Autodesk Inventor part; units mm, degrees
(part 2 of 2)
sketch "Sketch20" plane through (0, 0, 1) normal (0, 0, -1) x (-1, 0, 0)
  circle A0 centre (13.284, -4.42) radius 2.05 projected
  circle A1 centre (-13.284, 4.42) radius 2.05 projected
  circle A2 centre (-2.8142, 13.7142) radius 2.05 projected
  circle A3 centre (2.8142, -13.7142) radius 2.05 projected
  circle A4 centre (-10.4698, -9.2943) radius 2.05 projected
  circle A5 centre (10.4698, 9.2943) radius 2.05 projected
  arc A6 (-16.9842, 20.9889) -> (18.8277, -19.3525) centre (0, 0) ccw projected
  line L0 (18.8277, -19.3525) -> (17.641, -18.1327) projected
  arc A7 (16.8781, -10.7298) -> (17.641, -18.1327) centre (21.9416, -13.9488) ccw projected
  arc A8 (16.8781, -10.7298) -> (-8.6535, 18.031) centre (0, 0) ccw projected
  arc A9 (-15.9137, 19.666) -> (-8.6535, 18.031) centre (-11.2495, 23.4403) ccw projected
  line L1 (-15.9137, 19.666) -> (-16.9842, 20.9889) projected
  circle A10 centre (0, 0) radius 8.075 projected
  circle A11 centre (0, 0) radius 20
  circle A12 centre (-25.0527, -22.2399) radius 2.05 projected
  circle A13 centre (-31.7866, 10.5764) radius 2.05 projected
  circle A14 centre (-31.7866, 10.5764) radius 2.05 projected
  line L2 (0, 0) -> (-31.7866, 10.5764)
  circle A15 centre (-25.0527, -22.2399) radius 2.05 projected
  line L3 (0, 0) -> (-25.0527, -22.2399)
  line L4 (0, 0) -> (-25.7367, -8.1623)
  arc A16 (-16.9842, 20.9889) -> (18.8277, -19.3525) centre (0, 0) ccw projected
  point P0 (-25.7367, -8.1623)
  point P1 (-19.0642, -6.0461)
  point P2 (-18.9771, 6.3143)
  point P3 (-25.6191, 8.5242)
  dimension "d87" = 40
  dimension "d88" = 24
  constraints: 6 end point, 1 centre point, 1 coincident, 1 point on circle
  measures "d87" diameter of A11
  measures "d88" angle of L3 L4
extrude "Extrusion19" cut sketch "Sketch20" against normal blind 10 contours A11 L4 A6 L2
fillet "Fillet6" radius 2 4 edges at (25.7367, -8.1623, 3.5) (25.6191, 8.5242, 3.5) (18.9771, 6.3143, 3.5) (19.0642, -6.0461, 3.5)
ref_plane "Work Plane8" through (135.6695, -123.0192, -2.2) normal (0.6717255, 0.7408001, 0) x (0, 0, 1)
mirror "Mirror1" about plane through (135.6695, -123.0192, -2.2) normal (0.6717255, 0.7408001, 0) of "Extrusion19", "Fillet6"
sketch "Sketch21" plane through (0, 0, 1) normal (0, 0, -1) x (-1, 0, 0)
  circle A0 centre (-10.4698, -9.2943) radius 2.05 projected
  line L0 (0, 0) -> (-10.4698, -9.2943)
  line L1 (-10.4698, -9.2943) -> (-17.5743, -15.6011)
  circle A1 centre (-17.5743, -15.6011) radius 2.05
  dimension "d92" = 9.5
  dimension "d93" = 4.1
  constraints: 4 end point, 1 centre point, 1 coincident, 1 point on line
  measures "d92" distance of L0.end L1.end
  measures "d93" diameter of A1
extrude "Extrusion20" cut sketch "Sketch21" against normal blind 10 contours A1
body "Solid1"
